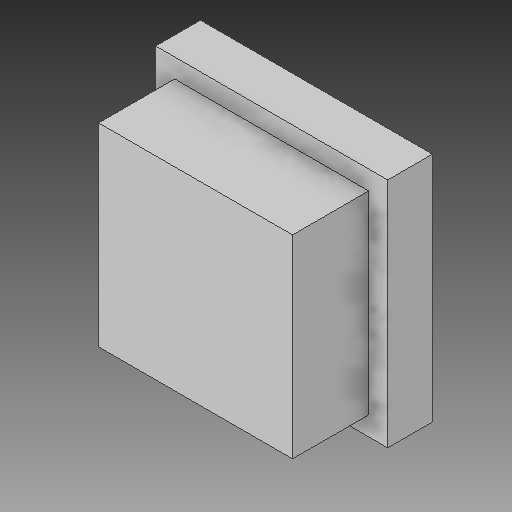
# Autodesk Inventor part: Circuit_OKL-T3-W12N-C
Saved by Autodesk Inventor 2018.2 (Build 222227000, 227)
## iProperties
Created: 2018-02-16
Part Number: Circuit_OKL-T3-W12N-C
Material: 一般
Document SubType Name: Modeling
Designer: sktom
Density: 1 g/cm^3
Appearance: 既定
Author: sktom
Autodesk Inventor part; units mm, degrees
ref_plane "YZ Plane" through (0, 0, 0) normal (1, 0, 0) x (0, 1, 0)
ref_plane "XZ Plane" through (0, 0, 0) normal (0, 1, 0) x (-1, 0, 0)
ref_plane "XY Plane" through (0, 0, 0) normal (0, 0, 1) x (1, 0, 0)
sketch "スケッチ1" plane through (0, 0, 0) normal (0, 0, 1) x (1, 0, 0)
  line L0 (-6.095, 6.095) -> (6.095, 6.095)
  line L1 (6.095, 6.095) -> (6.095, -6.095)
  line L2 (6.095, -6.095) -> (-6.095, -6.095)
  line L3 (-6.095, -6.095) -> (-6.095, 6.095)
  line L4 (-6.095, 6.095) -> (6.095, -6.095) construction
  line L5 (6.095, 6.095) -> (-6.095, -6.095) construction
  point P0 (0, 0)
  dimension "d0" = 12.19
  dimension "d1" = 12.19
  constraints: 12 end point, 2 midpoint, 2 parallel, 1 horizontal, 1 perpendicular
  measures "d0" distance of L0.start L0.end
  measures "d1" distance of L0.end L1.end
extrude "押し出し1" add sketch "スケッチ1" along normal blind 6.35
sketch "スケッチ2" plane through (0, 0, 6.35) normal (0, 0, 1) x (1, 0, 0)
  line L0 (6.095, 6.095) -> (-6.095, 6.095) projected
  line L1 (-6.095, -6.095) -> (6.095, -6.095)
  line L2 (6.095, -6.095) -> (6.095, 6.095)
  line L3 (6.095, 6.095) -> (-6.095, 6.095)
  line L4 (-6.095, 6.095) -> (-6.095, -6.095)
  line L5 (-6.095, -6.095) -> (6.095, 6.095) construction
  line L6 (6.095, -6.095) -> (-6.095, 6.095) construction
  line L7 (-5.095, -5.095) -> (5.095, -5.095)
  line L8 (5.095, -5.095) -> (5.095, 5.095)
  line L9 (5.095, 5.095) -> (-5.095, 5.095)
  line L10 (-5.095, 5.095) -> (-5.095, -5.095)
  point P0 (0, 0)
  dimension "d4" = 1
  constraints: 20 end point, 4 parallel, 2 midpoint, 2 perpendicular, 1 horizontal, 3 other
  measures "d4" distance between parallel lines of L4 L10
extrude "押し出し2" cut sketch "スケッチ2" against normal blind 4
